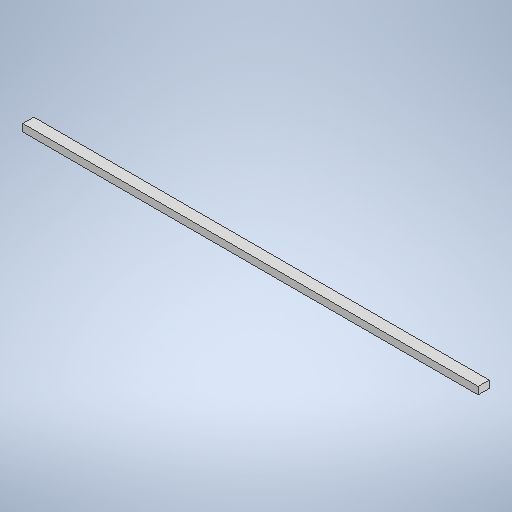
# Autodesk Inventor part: Rail 3.75x150
Saved by Autodesk Inventor 2025 (Build 290162000, 162)
## iProperties
Created: 2024-07-03
Part Number: Rail 3.75x150
Material: Generic
Document SubType Name: Modeling
Designer: adam
Density: 1 g/cm^3
Appearance: Default
Author: adam
Autodesk Inventor part; units mm, degrees
ref_plane "YZ Plane" through (0, 0, 0) normal (1, 0, 0) x (0, 1, 0)
ref_plane "XZ Plane" through (0, 0, 0) normal (0, 1, 0) x (-1, 0, 0)
ref_plane "XY Plane" through (0, 0, 0) normal (0, 0, 1) x (1, 0, 0)
sketch "Sketch1" plane through (0, 0, 0) normal (0, 0, 1) x (1, 0, 0)
  line L0 (0, 0) -> (155, 0)
  line L1 (155, 0) -> (155, -2.5)
  line L2 (155, -2.5) -> (0, -2.5)
  line L3 (0, -2.5) -> (0, 0)
  dimension "d0" = 2.5
  dimension "d1" = 155
  constraints: 8 end point, 2 parallel, 1 horizontal, 1 perpendicular
  measures "d0" distance of L2.end L0.start
  measures "d1" distance of L1.end L2.end
extrude "Extrusion1" add sketch "Sketch1" along normal blind 3.75
body "Solid1"
